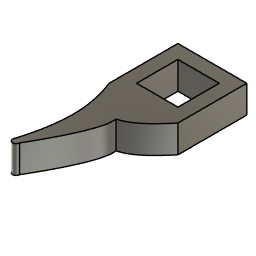
top part (Autodesk Fusion 360 design; units mm, degrees)
Autodesk Fusion 360 part; units mm, degrees
sketch "Sketch1" plane through (0, 0, 0) normal (0, 0, 1) x (1, 0, 0)
  line L0 (50, 150) -> (100, 150)
  line L1 (100, 150) -> (100, 100)
  line L2 (50, 100) -> (50, 150)
  spline S0 degree 5 poles (100, 100) (99.4525, 99.3417) (98.3613, 98.0463) (96.7361, 96.1664) (94.5929, 93.7883) (91.9562, 91.0458) (89.3665, 88.5583) (86.8289, 86.3543) (84.3485, 84.4604) (81.927, 82.8868) (79.5619, 81.6202) (77.7123, 80.8371) (76.3476, 80.3718) (75.4475, 80.115) (75, 80) knots 0 0 0 0 0 0 0.1 0.2 0.3 0.4 0.5 0.6 0.7 0.8 0.9 1 1 1 1 1 1
  spline S1 degree 5 poles (55, 30) (56.1485, 31.9792) (58.3768, 35.8759) (61.5128, 41.5355) (65.2748, 48.7047) (69.2207, 56.9863) (72.3132, 64.5009) (74.3236, 70.8187) (75.1164, 75.0951) (75.2245, 77.8092) (75.0941, 79.3618) (75, 80) knots 0 0 0 0 0 0 0.1 0.2 0.3 0.4 0.5 0.6 0.676319 0.676319 0.676319 0.676319 0.676319 0.676319
  line L3 (75.4166, 77.1741) -> (74.5834, 82.8259)
  arc A0 (50.4329, 31.406) -> (55, 30) centre (52.5, 30) ccw
  spline S2 degree 5 poles (50, 100) (50.4968, 98.7456) (51.4461, 96.2239) (52.7369, 92.4022) (54.1873, 87.2274) (55.5197, 80.6179) (56.3318, 73.856) (56.5867, 66.9307) (56.2741, 59.839) (55.4266, 52.5906) (54.138, 45.4687) (52.7912, 39.7298) (51.6306, 35.4454) (50.8139, 32.6619) (50.4329, 31.406) knots 0 0 0 0 0 0 0.1 0.2 0.3 0.4 0.5 0.6 0.7 0.8 0.9 0.981726 0.981726 0.981726 0.981726 0.981726 0.981726
  line L4 (52.6247, 38.6303) -> (48.241, 24.1818)
  line L5 (60, 140) -> (90, 140)
  line L6 (90, 140) -> (90, 110)
  line L7 (90, 110) -> (60, 110)
  line L8 (60, 110) -> (60, 140)
  point P0 (56.4359, 68.5598)
  point P1 (85, 85)
  constraint horizontal L0
  constraint vertical L1
  constraint vertical L2
  constraint midpoint S0.end L3
  constraint midpoint A0.start L4
  constraint horizontal L5
  constraint vertical L6
  constraint horizontal L7
  constraint vertical L8
extrude "Extrude1" add sketch "Sketch1" along normal blind 20
